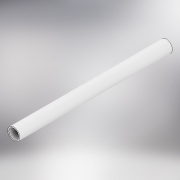
# Autodesk Inventor part: Tubo6
Saved by Autodesk Inventor 2021 (Build 250183000, 183)
## iProperties
Created: 2024-02-22
Part Number: Tubo6
Material: PVC-Piping
Document SubType Name: Modeling
Designer: Martin
Density: 1.4 g/cm^3
Appearance: Smooth - White
Mass: 19.0406 g
Surface Area: 176.877 cm^2
Volume: 13.6004 cm^3
Author: Martin
Autodesk Inventor part; units mm, degrees
ref_plane "YZ Plane" through (0, 0, 0) normal (1, 0, 0) x (0, 1, 0)
ref_plane "XZ Plane" through (0, 0, 0) normal (0, 1, 0) x (-1, 0, 0)
ref_plane "XY Plane" through (0, 0, 0) normal (0, 0, 1) x (1, 0, 0)
sketch "Sketch1" plane through (0, 0, 0) normal (0, 0, 1) x (1, 0, 0)
  circle A0 centre (0, 0) radius 6.35
  circle A1 centre (0, 0) radius 7.9
  dimension "d0" = 12.7
  dimension "d1" = 15.8
  constraints: 2 centre point, 2 coincident
  measures "d0" diameter of A0
  measures "d1" diameter of A1
extrude "Extrusion1" add sketch "Sketch1" along normal blind 196
body "Solid1"
